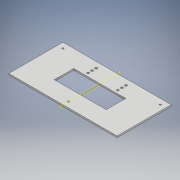
# Autodesk Inventor part: Up Base
Saved by Autodesk Inventor 2018 (Build 220112000, 112)
## iProperties
Created: 2020-02-13
Part Number: Up Base
Material: Типовые
Document SubType Name: Modeling
Designer: cosko
Density: 1 g/cm^3
Appearance: По умолчанию
Author: cosko
Autodesk Inventor part; units mm, degrees
ref_plane "YZ Plane" through (0, 0, 0) normal (1, 0, 0) x (0, 1, 0)
ref_plane "XZ Plane" through (0, 0, 0) normal (0, 1, 0) x (-1, 0, 0)
ref_plane "XY Plane" through (0, 0, 0) normal (0, 0, 1) x (1, 0, 0)
sketch "Эскиз1" plane through (0, 0, 0) normal (0, 0, 1) x (1, 0, 0)
  line L0 (-100, -50) -> (100, -50)
  line L1 (100, -50) -> (100, 50)
  line L2 (100, 50) -> (-100, 50)
  line L3 (-100, 50) -> (-100, -50)
  line L4 (-100, -50) -> (100, 50) construction
  line L5 (100, -50) -> (-100, 50) construction
  line L6 (-45, -15) -> (45, -15) construction
  line L7 (45, -15) -> (45, 15) construction
  line L8 (45, 15) -> (-45, 15) construction
  line L9 (-45, 15) -> (-45, -15) construction
  line L10 (-45, -15) -> (45, 15) construction
  line L11 (45, -15) -> (-45, 15) construction
  line L12 (0, 15) -> (0, 18) construction
  line L13 (-45, 15) -> (-48, 15) construction
  line L14 (48, -18) -> (-48, -18)
  line L15 (-48, -18) -> (-48, 18)
  line L16 (-48, 18) -> (48, 18)
  line L17 (48, 18) -> (48, -18)
  line L18 (48, -18) -> (-48, 18) construction
  line L19 (-48, -18) -> (48, 18) construction
  point P0 (0, 0)
  dimension "d0" = 200
  dimension "d1" = 100
  dimension "d2" = 90
  dimension "d3" = 30
  dimension "d4" = 3
  dimension "d5" = 3
  constraints: 40 end point, 7 midpoint, 6 parallel, 4 horizontal, 3 perpendicular, 1 vertical
  measures "d0" distance of L2.end L1.end
  measures "d1" distance of L1.end L0.end
  measures "d2" distance of L8.end L7.end
  measures "d3" distance of L7.end L6.end
  measures "d4" distance of L12.start L12.end
  measures "d5" distance of L8.end L13.end
extrude "Выдавливание1" add sketch "Эскиз1" along normal blind 3
ref_plane "РабПлоскость1" through (0, -50, 0) normal (1, 0, 0) x (0, 0, -1)
sketch "Эскиз2" plane through (0, 0, 3) normal (0, 0, 1) x (1, 0, 0)
  line L0 (-48, -18) -> (-48, 18) projected
  line L1 (-48, 18) -> (48, 18) projected
  line L2 (48, 18) -> (48, -18) projected
  line L3 (48, -18) -> (-48, -18) projected
  line L4 (-100, -50) -> (100, -50) projected
  line L5 (100, -50) -> (100, 50) projected
  line L6 (100, 50) -> (-100, 50) projected
  line L7 (-100, 50) -> (-100, -50) projected
  line L8 (48, 18) -> (33.5, 18) construction
  line L9 (33.5, 18) -> (33.5, 50) construction
  line L10 (33.5, 18) -> (27.5, 18) construction
  line L11 (48, 18) -> (-48, 18) construction
  line L12 (27.5, 18) -> (27.5, 50) construction
  line L13 (100, 50) -> (-100, 50) construction
  line L14 (27.5, 18) -> (27.5, 24) construction
  circle A0 centre (27.5, 24) radius 2
  circle A1 centre (27.5, 31.5) radius 2
  circle A2 centre (27.5, 39) radius 2
  line L15 (0, 18) -> (0, 50)
  line L16 (-33.5, 18) -> (-27.5, 18) construction
  line L17 (-27.5, 18) -> (-27.5, 24) construction
  circle A3 centre (-27.5, 24) radius 2
  circle A4 centre (-27.5, 31.5) radius 2
  circle A5 centre (-27.5, 39) radius 2
  point P0 (0, 0)
  dimension "d8" = 14.5
  dimension "d9" = 6
  dimension "d10" = 6
  dimension "d11" = 4
  dimension "d14" = 7.5
  constraints: 16 end point, 6 centre point, 6 symmetric about line, 5 point on line, 2 coincident, 2 midpoint, 2 perpendicular, 1 vertical, 7 other
  measures "d8" distance of L1.end L8.end
  measures "d9" distance of L8.end L10.end
  measures "d10" distance of L10.end L14.end
  measures "d11" diameter of A0
  measures "d14" distance of A0.centre A1.centre
extrude "Выдавливание2" cut sketch "Эскиз2" against normal blind 10 contours A0 | A1 | A2 | A3 | A4 | A5
sketch "Эскиз3" plane through (0, 0, 3) normal (0, 0, 1) x (1, 0, 0)
  circle A0 centre (-27.5, 31.5) radius 2 projected
  circle A1 centre (27.5, 39) radius 2 projected
  circle A2 centre (27.5, 24) radius 2 projected
  circle A3 centre (27.5, 31.5) radius 2 projected
  circle A4 centre (-27.5, 24) radius 2 projected
  circle A5 centre (-27.5, 39) radius 2 projected
  line L0 (-48, -18) -> (-48, 18) projected
  line L1 (-48, 18) -> (48, 18) projected
  line L2 (48, 18) -> (48, -18) projected
  line L3 (48, -18) -> (-48, -18) projected
  line L4 (-100, -50) -> (100, -50) projected
  line L5 (100, -50) -> (100, 50) projected
  line L6 (100, 50) -> (-100, 50) projected
  line L7 (-100, 50) -> (-100, -50) projected
  line L8 (-100, 50) -> (-90, 50) construction
  line L9 (-90, 50) -> (-90, 40) construction
  line L10 (-90, 40) -> (-100, 40) construction
  line L11 (-100, 40) -> (-100, 50) construction
  circle A6 centre (-90, 40) radius 1.5
  line L12 (-100, 50) -> (-100, -50) projected
  line L13 (-100, 0) -> (100, 0)
  line L14 (100, -50) -> (100, 50) projected
  line L15 (100, 50) -> (-100, 50) projected
  line L16 (0, 50) -> (0, -50)
  line L17 (-100, -50) -> (100, -50) projected
  circle A7 centre (90, 40) radius 1.5
  line L18 (0, -50) -> (0, -40) construction
  circle A8 centre (0, -40) radius 1.5
  point P0 (0, 0)
  dimension "d21" = 10
  dimension "d22" = 10
  dimension "d23" = 3
  dimension "d24" = 10
  dimension "d25" = 3
  constraints: 14 end point, 4 midpoint, 3 centre point, 3 coincident, 2 parallel, 2 symmetric about line, 1 horizontal, 1 perpendicular, 1 point on line, 1 other
  measures "d21" distance of L9.end L10.end
  measures "d22" distance of L8.end L9.end
  measures "d23" diameter of A6
  measures "d24" distance of L16.end L18.end
  measures "d25" diameter of A8
extrude "Выдавливание3" cut sketch "Эскиз3" against normal blind 10 contours A8 L16 | L16 A8 | A6 | A7
